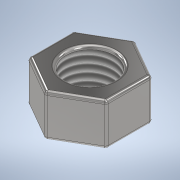
# Autodesk Inventor part: M3_12mm
Saved by Autodesk Inventor 2021 (Build 250183000, 183)
## iProperties
Created: 2021-07-23
Part Number: M3_12mm
Material: Generic
Document SubType Name: Modeling
Designer: zmac845
Density: 1 g/cm^3
Appearance: Steel - Polished
Author: zmac845
Autodesk Inventor part; units mm, degrees
ref_plane "YZ Plane" through (0, 0, 0) normal (1, 0, 0) x (0, 1, 0)
ref_plane "XZ Plane" through (0, 0, 0) normal (0, 1, 0) x (-1, 0, 0)
ref_plane "XY Plane" through (0, 0, 0) normal (0, 0, 1) x (1, 0, 0)
sketch "Sketch1" plane through (0, 0, 0) normal (0, 1, 0) x (-1, 0, 0)
  circle A0 centre (0, 0) radius 4
  line L0 (6.5, 3.7528) -> (6.5, -3.7528)
  line L1 (6.5, -3.7528) -> (0, -7.5056)
  line L2 (0, -7.5056) -> (-6.5, -3.7528)
  line L3 (-6.5, -3.7528) -> (-6.5, 3.7528)
  line L4 (-6.5, 3.7528) -> (0, 7.5056)
  line L5 (0, 7.5056) -> (6.5, 3.7528)
  dimension "d0" = 8
  dimension "d9" = 13
  constraints: 12 end point, 2 coincident, 1 centre point, 1 vertical, 13 other
  measures "d0" diameter of A0
  measures "d9" distance between parallel lines of L3 L0
extrude "Extrusion3" add sketch "Sketch1" along normal blind 7
fillet "Fillet2" radius 0.5 20 edges at (0, 3.5, 7.5056) (6.5, 3.5, 3.7528) (3.25, 0, 5.6292) (6.5, 0, 0) (6.5, 3.5, -3.7528) (6.5, 7, 0) (3.25, 7, -5.6292) (-3.25, 7, -5.6292) (-6.5, 7, 0) (-3.25, 7, 5.6292) (3.25, 7, 5.6292) (-3.25, 0, 5.6292) (-6.5, 3.5, 3.7528) (-6.5, 3.5, -3.7528) (0, 3.5, -7.5056) (-3.25, 0, -5.6292) (3.25, 0, -5.6292) (-6.5, 0, 0) (4, 7, 0) (4, 0, 0)
thread "Thread2" size "M8x1.25" class "6H" standard "ANSI Metric M Profile" full length
body "Solid2"
